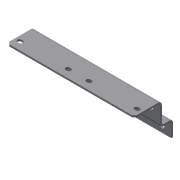
# Autodesk Inventor part: Bearing Base
Saved by Autodesk Inventor 2016 (Build 200138000, 138)
## iProperties
Created: 2012-10-11
Part Number: Bearing Base
Material: Generic
Document SubType Name: Sheet Metal
Designer: bruno.silveira
Density: 1 g/cm^3
Sheet Metal Rule: Default_mm
Appearance: Default
Mass: 1333.01 g
Surface Area: 3531.75 cm^2
Volume: 1333.01 cm^3
Author: bruno.silveira
Autodesk Inventor part; units mm, degrees
ref_plane "YZ Plane" through (0, 0, 0) normal (1, 0, 0) x (0, 1, 0)
ref_plane "XZ Plane" through (0, 0, 0) normal (0, 1, 0) x (-1, 0, 0)
ref_plane "XY Plane" through (0, 0, 0) normal (0, 0, 1) x (1, 0, 0)
sketch "Sketch1" plane through (0, 0, 0) normal (0, 0, 1) x (1, 0, 0)
  line L0 (0, 0) -> (555, 0)
  line L1 (555, 0) -> (555, 120)
  line L2 (555, 120) -> (0, 120)
  line L3 (0, 120) -> (0, 0)
  dimension "d0" = 120
  dimension "d1" = 555
  measures "d0" distance of L2.end L0.start
  measures "d1" distance of L0.start L0.end
extrude "Plate1" add sketch "Sketch1" along normal blind 8
sketch "Sketch2" plane through (555, 112, 8) normal (0, 1, 0) x (-1, 0, 0)
  line L0 (555, 0) -> (0, 0)
  line L1 (0, 0) -> (0, -100)
  line L2 (0, -100) -> (555, -100)
  line L3 (555, -100) -> (555, 0)
  constraints: 6 end point, 1 horizontal, 1 perpendicular, 1 vertical
edge flange "Flange1" height 100 angle 90 thickness 8 bend radius 8 thickness toward (0, 1, 0) relief tear relief width 8 relief depth 4 edges at (277.5, 120, 0) wall of the first edge with corners at (0, 112, 8) (555, 112, 8) (555, 112, -92) (0, 112, -92)
bend "Bend1"
corner "Corner1"
sketch "Sketch3" plane through (0, 112, -92) normal (0, -1, 0) x (1, 0, 0)
  line L0 (0, 0) -> (0, 84) projected
  line L1 (0, 0) -> (555, 0) projected
  line L2 (555, 0) -> (555, 84) projected
  circle A0 centre (40, 60) radius 10
  circle A1 centre (515, 60) radius 10
  circle A2 centre (220, 60) radius 10
  circle A3 centre (335, 60) radius 10
  point P0 (0, 92)
  dimension "d13" = 20
  dimension "d14" = 20
  dimension "d15" = 40
  dimension "d16" = 60
  dimension "d17" = 60
  dimension "d18" = 40
  dimension "d19" = 20
  dimension "d20" = 180
  dimension "d21" = 20
  dimension "d22" = 180
  dimension "d23" = 60
  dimension "d24" = 60
  constraints: 4 centre point
  measures "d13" diameter of A0
  measures "d14" diameter of A1
  measures "d15" distance from line of L0 A0.centre
  measures "d16" distance from line of L1 A0.centre
  measures "d17" distance from line of L1 A1.centre
  measures "d18" distance from line of L2 A1.centre
  measures "d19" diameter of A2
  measures "d20" distance of A0.centre A2.centre
  measures "d21" diameter of A3
  measures "d22" distance of A1.centre A3.centre
  measures "d23" distance from line of L1 A3.centre
  measures "d24" distance from line of L1 A2.centre
hole "Hole1" at (40, 112, -32) at (220, 112, -32) at (335, 112, -32) at (515, 112, -32) direction (0, 1, 0) diameter 20 depth 8 tip angle 118
sketch "Sketch4" plane through (0, 0, 8) normal (0, 0, 1) x (1, 0, 0)
  circle A0 centre (544.5, 10.5) radius 1.1625 projected
  circle A1 centre (544.5, 59.5) radius 1.1625 projected
  arc A2 (535.5, 26) -> (535.5, 44) centre (535.5, 35) ccw projected
  line L0 (535.5, 26) -> (529.5, 26) projected
  arc A3 (529.5, 44) -> (529.5, 26) centre (529.5, 35) ccw projected
  line L1 (529.5, 44) -> (535.5, 44) projected
  line L2 (507.5, 26.468) -> (507.5, 43.532) projected
  arc A4 (505.7408, 21) -> (507.5, 26.468) centre (471.6029, 35) ccw projected
  line L3 (505.7408, 21) -> (482.22, 0) projected
  line L4 (482.22, 0) -> (545, 0) projected
  line L5 (545, 0) -> (553, 8) projected
  line L6 (553, 8) -> (553, 62) projected
  line L7 (553, 62) -> (545, 70) projected
  line L8 (482.22, 70) -> (545, 70) projected
  line L9 (482.22, 70) -> (505.7408, 49) projected
  arc A5 (507.5, 43.532) -> (505.7408, 49) centre (471.6029, 35) ccw projected
  circle A6 centre (310.5, 10.5) radius 1.1625 projected
  circle A7 centre (310.5, 59.5) radius 1.1625 projected
  arc A8 (325.5, 26) -> (325.5, 44) centre (325.5, 35) ccw projected
  line L10 (325.5, 26) -> (319.5, 26) projected
  arc A9 (319.5, 44) -> (319.5, 26) centre (319.5, 35) ccw projected
  line L11 (319.5, 44) -> (325.5, 44) projected
  line L12 (347.5, 26.468) -> (347.5, 43.532) projected
  arc A10 (349.2592, 49) -> (347.5, 43.532) centre (383.3971, 35) ccw projected
  line L13 (349.2592, 49) -> (372.78, 70) projected
  line L14 (372.78, 70) -> (310, 70) projected
  line L15 (310, 70) -> (302, 62) projected
  line L16 (302, 8) -> (302, 62) projected
  line L17 (302, 8) -> (310, 0) projected
  line L18 (372.78, 0) -> (310, 0) projected
  line L19 (372.78, 0) -> (349.2592, 21) projected
  arc A11 (347.5, 26.468) -> (349.2592, 21) centre (383.3971, 35) ccw projected
  circle A12 centre (244.5, 10.5) radius 1.1625 projected
  circle A13 centre (244.5, 59.5) radius 1.1625 projected
  arc A14 (235.5, 26) -> (235.5, 44) centre (235.5, 35) ccw projected
  line L20 (235.5, 26) -> (229.5, 26) projected
  arc A15 (229.5, 44) -> (229.5, 26) centre (229.5, 35) ccw projected
  line L21 (229.5, 44) -> (235.5, 44) projected
  line L22 (207.5, 26.468) -> (207.5, 43.532) projected
  arc A16 (205.7408, 21) -> (207.5, 26.468) centre (171.6029, 35) ccw projected
  line L23 (205.7408, 21) -> (182.22, 0) projected
  line L24 (182.22, 0) -> (245, 0) projected
  line L25 (245, 0) -> (253, 8) projected
  line L26 (253, 8) -> (253, 62) projected
  line L27 (253, 62) -> (245, 70) projected
  line L28 (182.22, 70) -> (245, 70) projected
  line L29 (182.22, 70) -> (205.7408, 49) projected
  arc A17 (207.5, 43.532) -> (205.7408, 49) centre (171.6029, 35) ccw projected
  circle A18 centre (10.5, 10.5) radius 1.1625 projected
  circle A19 centre (10.5, 59.5) radius 1.1625 projected
  arc A20 (25.5, 26) -> (25.5, 44) centre (25.5, 35) ccw projected
  line L30 (25.5, 26) -> (19.5, 26) projected
  arc A21 (19.5, 44) -> (19.5, 26) centre (19.5, 35) ccw projected
  line L31 (19.5, 44) -> (25.5, 44) projected
  line L32 (47.5, 26.468) -> (47.5, 43.532) projected
  arc A22 (49.2592, 49) -> (47.5, 43.532) centre (83.3971, 35) ccw projected
  line L33 (49.2592, 49) -> (72.78, 70) projected
  line L34 (72.78, 70) -> (10, 70) projected
  line L35 (10, 70) -> (2, 62) projected
  line L36 (2, 8) -> (2, 62) projected
  line L37 (2, 8) -> (10, 0) projected
  line L38 (72.78, 0) -> (10, 0) projected
  line L39 (72.78, 0) -> (49.2592, 21) projected
  arc A23 (47.5, 26.468) -> (49.2592, 21) centre (83.3971, 35) ccw projected
extrude "Extrusion1" cut sketch "Sketch4" against normal blind 10 contours L0 A3 L1 A2 | L10 A9 L11 A8 | L20 A15 L21 A14 | L30 A21 L31 A20
chamfer "Corner Chamfer1" distance 10 angle 45 2 edges at (555, 0, 4) (0, 0, 4)
sketch "Sketch5" plane through (0, 112, -84) normal (0, 0, -1) x (-1, 0, 0)
  line L0 (-555, 0) -> (0, 0)
  line L1 (0, 0) -> (0, 57)
  line L2 (0, 57) -> (-555, 57)
  line L3 (-555, 57) -> (-555, 0)
  constraints: 6 end point, 1 horizontal, 1 perpendicular, 1 vertical
edge flange "Flange2" height 57 angle 90 thickness 8 bend radius 8 thickness toward (0, 0, -1) relief tear relief width 8 relief depth 4 edges at (277.5, 120, -92) wall of the first edge with corners at (555, 112, -84) (0, 112, -84) (0, 169, -84) (555, 169, -84)
bend "Bend2"
corner "Corner2"
sketch "Sketch6" plane through (555, 161, -84) normal (0, 1, 0) x (-1, 0, 0)
  line L0 (555, 0) -> (0, 0)
  line L1 (0, 0) -> (0, -70)
  line L2 (0, -70) -> (555, -70)
  line L3 (555, -70) -> (555, 0)
  constraints: 6 end point, 1 horizontal, 1 perpendicular, 1 vertical
edge flange "Flange3" height 70 angle 90 thickness 8 bend radius 8 thickness toward (0, 1, 0) relief tear relief width 8 relief depth 4 edges at (277.5, 169, -92) wall of the first edge with corners at (0, 161, -84) (555, 161, -84) (555, 161, -154) (0, 161, -154)
bend "Bend3"
corner "Corner3"
sketch "Sketch7" plane through (0, 161, -154) normal (0, -1, 0) x (1, 0, 0)
  line L0 (0, 0) -> (0, 54) projected
  line L1 (0, 0) -> (555, 0) projected
  line L2 (555, 0) -> (555, 54) projected
  circle A0 centre (40, 27) radius 10
  circle A1 centre (515, 27) radius 10
  circle A2 centre (220, 27) radius 10
  circle A3 centre (335, 27) radius 10
  point P0 (0, 154)
  dimension "d57" = 20
  dimension "d58" = 40
  dimension "d59" = 27
  dimension "d60" = 20
  dimension "d61" = 40
  dimension "d62" = 27
  dimension "d63" = 20
  dimension "d64" = 20
  dimension "d65" = 180
  dimension "d66" = 27
  dimension "d67" = 180
  dimension "d68" = 27
  constraints: 4 centre point
  measures "d57" diameter of A0
  measures "d58" distance from line of L0 A0.centre
  measures "d59" distance from line of L1 A0.centre
  measures "d60" diameter of A1
  measures "d61" distance from line of L2 A1.centre
  measures "d62" distance from line of L1 A1.centre
  measures "d63" diameter of A2
  measures "d64" diameter of A3
  measures "d65" distance of A0.centre A2.centre
  measures "d66" distance from line of L1 A2.centre
  measures "d67" distance of A1.centre A3.centre
  measures "d68" distance from line of L1 A3.centre
hole "Hole2" at (40, 161, -127) at (220, 161, -127) at (335, 161, -127) at (515, 161, -127) direction (0, 1, 0) diameter 20 depth 8 tip angle 118
equation "\"d30\" = Thickness"
equation "\"d74\" = Thickness"
equation "\"d3\" = BendReliefWidth"
equation "\"d4\" = BendReliefDepth"
equation "\"d5\" = MinimumRemnant"
equation "\"d6\" = BendRadius"
equation "\"d9\" = BendRadius"
equation "\"d10\" = CornerReliefSize"
equation "\"d11\" = GapSize"
equation "\"d12\" = JacobiRadiusSize"
equation "\"d37\" = BendReliefWidth"
equation "\"d38\" = BendReliefDepth"
equation "\"d39\" = MinimumRemnant"
equation "\"d40\" = BendRadius"
equation "\"d43\" = BendRadius"
equation "\"d44\" = CornerReliefSize"
equation "\"d45\" = GapSize"
equation "\"d46\" = JacobiRadiusSize"
equation "\"d47\" = BendReliefWidth"
equation "\"d48\" = BendReliefDepth"
equation "\"d49\" = MinimumRemnant"
equation "\"d50\" = BendRadius"
equation "\"d53\" = BendRadius"
equation "\"d54\" = CornerReliefSize"
equation "\"d55\" = GapSize"
equation "\"d56\" = JacobiRadiusSize"
equation "\"BendRadius\" = Thickness"
equation "\"BendReliefWidth\" = Thickness"
equation "\"BendReliefDepth\" = 0.5 * Thickness"
equation "\"CornerReliefSize\" = 4 * Thickness"
equation "\"MinimumRemnant\" = 2 * Thickness"
equation "\"TransitionRadius\" = BendRadius"
equation "\"JacobiRadiusSize\" = BendRadius"
equation "\"GapSize\" = Thickness"
equation "\"d2\" = BendRadius"
equation "\"Thickness\" = 8"
body "Solid1"
